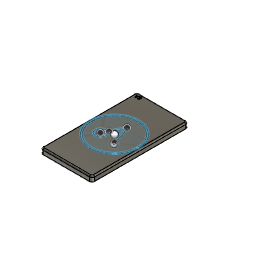
Top Box(V3) (Autodesk Fusion 360 design; units mm, degrees)
Autodesk Fusion 360 part; units mm, degrees
sketch "Sketch9" plane through (0, 0, 31.5) normal (0, 0, 1) x (-1, 0, 0)
  line L0 (-78, -4) -> (-78, -146)
  arc A0 (-78, -146) -> (-76, -148) centre (-76, -146) ccw
  line L1 (-76, -148) -> (-4, -148)
  arc A1 (-4, -148) -> (-2, -146) centre (-4, -146) ccw
  line L2 (-2, -146) -> (-2, -4)
  arc A2 (-2, -4) -> (-4, -2) centre (-4, -4) ccw
  line L3 (-4, -2) -> (-76, -2)
  arc A3 (-76, -2) -> (-78, -4) centre (-76, -4) ccw
  circle A4 centre (-40.047, -74.8176) radius 37.5
sketch "Sketch1" plane through (0, 0, 24) normal (0, 0, 1) x (-1, 0, 0)
  line L0 (-2, -4) -> (-2, -146)
  arc A0 (-4, -148) -> (-2, -146) centre (-4, -146) ccw
  line L1 (-4, -148) -> (-76, -148)
  arc A1 (-78, -146) -> (-76, -148) centre (-76, -146) ccw
  line L2 (-78, -146) -> (-78, -4)
  arc A2 (-76, -2) -> (-78, -4) centre (-76, -4) ccw
  line L3 (-76, -2) -> (-4, -2)
  arc A3 (-2, -4) -> (-4, -2) centre (-4, -4) ccw
  arc A4 (-80, -146) -> (-76, -150) centre (-76, -146) ccw
  line L4 (-76, -150) -> (-4, -150)
  arc A5 (-4, -150) -> (0, -146) centre (-4, -146) ccw
  line L5 (0, -146) -> (0, -4)
  arc A6 (0, -4) -> (-4, 0) centre (-4, -4) ccw
  line L6 (-4, 0) -> (-76, 0)
  arc A7 (-76, 0) -> (-80, -4) centre (-76, -4) ccw
  line L7 (-80, -4) -> (-80, -146)
  arc A8 (-4, -148) -> (-2, -146) centre (-4, -146) ccw
  line L8 (-2, -146) -> (-2, -4)
  arc A9 (-2, -4) -> (-4, -2) centre (-4, -4) ccw
  line L9 (-4, -2) -> (-76, -2)
  arc A10 (-76, -2) -> (-78, -4) centre (-76, -4) ccw
  line L10 (-78, -4) -> (-78, -146)
  arc A11 (-78, -146) -> (-76, -148) centre (-76, -146) ccw
  line L11 (-76, -148) -> (-4, -148)
  line L12 (-76, -146) -> (-76, -4)
  line L13 (-76, -4) -> (-4, -4)
  line L14 (-4, -4) -> (-4, -146)
  line L15 (-4, -146) -> (-76, -146)
extrude "Extrude1" add sketch "Sketch1" along normal up to surface (5 mm away) contours A4 L4 A5 L5 A6 L6 A7 L7
sketch "Sketch2" plane through (0, 0, 29) normal (0, 0, 1) x (-1, 0, 0)
  arc A0 (-4, -148) -> (-2, -146) centre (-4, -146) ccw
  line L0 (-2, -146) -> (-2, -4)
  arc A1 (-2, -4) -> (-4, -2) centre (-4, -4) ccw
  line L1 (-4, -2) -> (-76, -2)
  arc A2 (-76, -2) -> (-78, -4) centre (-76, -4) ccw
  line L2 (-78, -4) -> (-78, -146)
  arc A3 (-78, -146) -> (-76, -148) centre (-76, -146) ccw
  line L3 (-76, -148) -> (-4, -148)
  line L4 (-76, -146) -> (-76, -4)
  line L5 (-76, -4) -> (-4, -4)
  line L6 (-4, -4) -> (-4, -146)
  line L7 (-4, -146) -> (-76, -146)
  arc A4 (-4, -148) -> (-2, -146) centre (-4, -146) ccw
  line L8 (-4, -148) -> (-76, -148)
  arc A5 (-78, -146) -> (-76, -148) centre (-76, -146) ccw
  line L9 (-78, -146) -> (-78, -4)
  arc A6 (-76, -2) -> (-78, -4) centre (-76, -4) ccw
  line L10 (-76, -2) -> (-4, -2)
  arc A7 (-2, -4) -> (-4, -2) centre (-4, -4) ccw
  line L11 (-2, -4) -> (-2, -146)
  arc A8 (-76, 0) -> (-80, -4) centre (-76, -4) ccw
  line L12 (-80, -4) -> (-80, -146)
  arc A9 (-80, -146) -> (-76, -150) centre (-76, -146) ccw
  line L13 (-76, -150) -> (-4, -150)
  arc A10 (-4, -150) -> (0, -146) centre (-4, -146) ccw
  line L14 (0, -146) -> (0, -4)
  arc A11 (0, -4) -> (-4, 0) centre (-4, -4) ccw
  line L15 (-4, 0) -> (-76, 0)
extrude "Extrude2" add sketch "Sketch2" along normal blind 2.5 contours A0 L0 A1 L1 A2 L2 A3 L3 A4 L8 A5 L9 A6 L10 A7 L11 | L4 L5 L6 L7 | A8 L12 A9 L13 A10 L14 A11 L15
sketch "Sketch4" plane through (0, 0, 31.5) normal (0, 0, 1) x (-1, 0, 0)
  line L0 (-4, 0) -> (-76, 0)
  arc A0 (-76, 0) -> (-80, -4) centre (-76, -4) ccw
  line L1 (-80, -4) -> (-80, -146)
  arc A1 (-80, -146) -> (-76, -150) centre (-76, -146) ccw
  line L2 (-76, -150) -> (-4, -150)
  arc A2 (-4, -150) -> (0, -146) centre (-4, -146) ccw
  line L3 (0, -146) -> (0, -4)
  arc A3 (0, -4) -> (-4, 0) centre (-4, -4) ccw
sketch "Logo" plane through (0, 0, 31.5) normal (0, 0, 1) x (1, 0, 0)
  line L0 (39.985, 93.2735) -> (49.8354, 63.9379)
  arc A0 (49.8354, 63.9379) -> (51.7314, 64.5746) centre (50.7834, 64.2563) ccw
  line L1 (51.7314, 64.5746) -> (41.881, 93.9101)
  arc A1 (41.881, 93.9101) -> (39.985, 93.2735) centre (40.933, 93.5918) ccw
  line L2 (40.933, 93.5918) -> (50.7834, 64.2563) construction
  line L3 (40.0292, 94.0197) -> (31.0416, 75.0379)
  arc A2 (31.0416, 75.0379) -> (32.8492, 74.182) centre (31.9454, 74.61) ccw
  line L4 (32.8492, 74.182) -> (41.8368, 93.1638)
  arc A3 (41.8368, 93.1638) -> (40.0292, 94.0197) centre (40.933, 93.5918) ccw
  line L5 (40.933, 93.5918) -> (31.9454, 74.61) construction
  circle A4 centre (52.0776, 61.8835) radius 3.6273
  circle A5 centre (27.1281, 65.91) radius 4.7922
  circle A6 centre (29.1413, 67.8513) radius 0.7643
  circle A7 centre (27.1281, 65.91) radius 6.0199
  circle A8 centre (27.1281, 65.91) radius 8.0916
  circle A9 centre (40.047, 74.8176) radius 37.5
  circle A10 centre (40.047, 74.8176) radius 35.5
  circle A11 centre (52.0776, 61.8835) radius 2
  point P0 (27.1281, 65.91)
  point P1 (52.0776, 61.8835)
  dimension "d120" = 2
  dimension "d121" = 2
  dimension "d240" = 75
  dimension "d241" = 71
  dimension "d242" = 4
  constraint tangent L0 A0
  constraint tangent A0 L1
  constraint parallel L0 L1
  constraint tangent L1 A1
  constraint tangent L0 A1
  constraint tangent L3 A2
  constraint tangent A2 L4
  constraint parallel L3 L4
  constraint tangent L4 A3
  constraint tangent L3 A3
  constraint coincident A1.centre L2.start
  constraint concentric A5 A7
  constraint concentric A5 A8
  constraint coincident P0 A5.centre
  constraint concentric A9 A10
  constraint concentric A4 A11
  measures "d120" diameter of A0
  measures "d121" diameter of A2
  measures "d240" diameter of A9
  measures "d241" diameter of A10
  measures "d242" diameter of A11
extrude "Extrude6" cut sketch "Logo" against normal blind 1
sketch "Camera Shape" plane through (0, 0, 29) normal (0, 0, 1) x (1, 0, 0)
  line L0 (39.6281, 80.36) -> (14.6281, 80.36)
  line L1 (14.6281, 80.36) -> (14.6281, 56.36)
  line L2 (14.6281, 56.36) -> (39.6281, 56.36)
  line L3 (39.6281, 56.36) -> (39.6281, 80.36)
  circle A0 centre (16.6281, 78.36) radius 0.9
  circle A1 centre (16.6281, 66.16) radius 0.9
  line L4 (27.1281, 80.36) -> (27.1281, 56.36) construction
  circle A2 centre (16.6281, 78.36) radius 2
  circle A3 centre (16.6281, 66.16) radius 2
  circle A4 centre (37.6281, 78.36) radius 0.9
  circle A5 centre (37.6281, 78.36) radius 2
  circle A6 centre (37.6281, 66.16) radius 2
  circle A7 centre (37.6281, 66.16) radius 0.9
  line L5 (31.3781, 70.16) -> (22.8781, 70.16)
  line L6 (22.8781, 70.16) -> (22.8781, 61.66)
  line L7 (22.8781, 61.66) -> (31.3781, 61.66)
  line L8 (31.3781, 61.66) -> (31.3781, 70.16)
  line L9 (31.3781, 70.16) -> (22.8781, 61.66) construction
  line L10 (22.8781, 70.16) -> (31.3781, 61.66) construction
  circle A8 centre (27.1281, 65.91) radius 3.7
  arc A9 (76, 2) -> (78, 4) centre (76, 4) ccw
  line L11 (76, 2) -> (4, 2)
  arc A10 (2, 4) -> (4, 2) centre (4, 4) ccw
  line L12 (2, 4) -> (2, 146)
  arc A11 (4, 148) -> (2, 146) centre (4, 146) ccw
  line L13 (4, 148) -> (76, 148)
  arc A12 (78, 146) -> (76, 148) centre (76, 146) ccw
  line L14 (78, 146) -> (78, 4)
  point P0 (27.1281, 65.91)
  dimension "d98" = 25
  dimension "d99" = 24
  dimension "d100" = 1.8
  dimension "d101" = 2
  dimension "d102" = 2
  dimension "d103" = 1.8
  dimension "d104" = 2
  dimension "d105" = 12.2
  dimension "d106" = 4
  dimension "d107" = 8.5
  dimension "d108" = 8.5
  dimension "d110" = 10.2
  dimension "d111" = 8.25
  dimension "d112" = 8.25
  dimension "d113" = 7.4
  dimension "d133" = 4
  constraint horizontal L0
  constraint vertical L1
  constraint horizontal L2
  constraint vertical L3
  constraint midpoint L0 L4.start
  constraint midpoint L2 L4.end
  constraint concentric A0 A2
  constraint concentric A1 A3
  constraint symmetric A0 L4 A4
  constraint symmetric A1 L4 A7
  constraint symmetric L4 A2 A5
  constraint symmetric L4 A3 A6
  constraint horizontal L5
  constraint vertical L6
  constraint horizontal L7
  constraint vertical L8
  constraint midpoint L10 P0
  constraint coincident P0 A8.centre
  measures "d98" distance of L0.start L0.end
  measures "d99" distance of L0.start L2.end
  measures "d100" diameter of A0
  measures "d101" distance of L0 A0.centre
  measures "d102" distance of L1 A0.centre
  measures "d103" diameter of A1
  measures "d104" distance of L1 A1.centre
  measures "d105" distance of A0.centre A1.centre
  measures "d106" diameter of A2
  measures "d107" distance of L5.start L5.end
  measures "d108" distance of L5.start L7.end
  measures "d110" distance of L0 L5
  measures "d111" distance of L3 L8
  measures "d112" distance of L1 L6
  measures "d113" diameter of A8
  measures "d133" diameter of A3
extrude "Extrude3" cut sketch "Camera Shape" along normal up to surface (2.5 mm away) contours A8
extrude "Extrude4" cut sketch "Camera Shape" along normal blind 0.1 contours L5 L6 L7 L8
extrude "Extrude5" add sketch "Camera Shape" against normal blind 3.2 contours A3 | A6 | A5 | A2
sketch "LED Hole" plane through (0, 0, 29) normal (0, 0, -1) x (1, 0, 0)
  circle A0 centre (16.6281, -78.36) radius 2
  circle A1 centre (37.6281, -78.36) radius 2
  line L0 (22.8781, -61.66) -> (31.3781, -61.66)
  line L1 (31.3781, -61.66) -> (31.3781, -70.16)
  line L2 (31.3781, -70.16) -> (22.8781, -70.16)
  line L3 (22.8781, -70.16) -> (22.8781, -61.66)
  arc A2 (78, -4) -> (76, -2) centre (76, -4) ccw
  line L4 (76, -2) -> (4, -2)
  arc A3 (4, -2) -> (2, -4) centre (4, -4) ccw
  line L5 (2, -4) -> (2, -146)
  arc A4 (2, -146) -> (4, -148) centre (4, -146) ccw
  line L6 (4, -148) -> (76, -148)
  arc A5 (76, -148) -> (78, -146) centre (76, -146) ccw
  line L7 (78, -146) -> (78, -4)
  circle A6 centre (37.6281, -66.16) radius 2
  circle A7 centre (16.6281, -66.16) radius 2
  circle A8 centre (52.0776, -61.8835) radius 1.7
  circle A9 centre (52.0776, -61.8835) radius 2.5
  point P0 (52.0776, -61.8835)
  dimension "d139" = 3.4
  dimension "d140" = 5
  constraint coincident P0 A8.centre
  measures "d139" diameter of A8
  measures "d140" diameter of A9
extrude "Extrude8" cut sketch "LED Hole" against normal up to surface (2.5 mm away) contours A8
extrude "Extrude9" add sketch "LED Hole" along normal blind 2 contours A9
fillet "Fillet1" radius 2 8 edges at (80, 75, 31.5) (78.8284, 148.8284, 31.5) (40, 150, 31.5) (1.1716, 148.8284, 31.5) (0, 75, 31.5) (1.1716, 1.1716, 31.5) (40, 0, 31.5) (78.8284, 1.1716, 31.5)
sketch "Sketch8" plane through (0, 0, 31.5) normal (0, 0, 1) x (1, 0, 0)
  line L0 (4, 137.6943) -> (15.2201, 137.6943) construction
  line L1 (15.2201, 137.6943) -> (15.2201, 146) construction
  line L2 (15.2201, 146) -> (4, 146) construction
  line L3 (4, 146) -> (4, 137.6943) construction
  point P0 (4, 146)
  dimension "d211" = 5
  text T0 "V3" font "Arial" height 5 align left top in box 11.2201 x 8.3057 at (4, 137.6943) x (1, 0) y (0, 1) spacing 1 kerned
  constraint coincident P0
extrude "Extrude11" cut sketch "Sketch8" against normal blind 1 text T0
move_face "OffsetFaces1" offset 0.5 1 faces at (1.3333, 51.3333, 24)
equation "d111 = d112"
